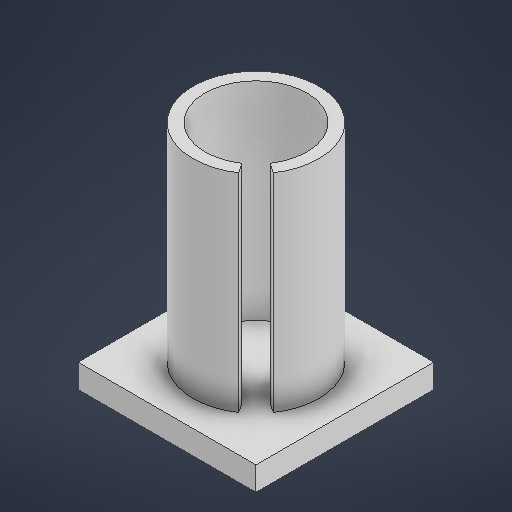
# Autodesk Inventor part: Część1
Saved by Autodesk Inventor 2026 (Build 300175050, 175E)
## iProperties
Created: 2026-01-10
Part Number: Część1
Material: Ogólny
Document SubType Name: Modeling
Designer: DeathLock
Density: 1 g/cm^3
Appearance: Domyślna
Author: DeathLock
Autodesk Inventor part; units mm, degrees
ref_plane "YZ Plane" through (0, 0, 0) normal (1, 0, 0) x (0, 1, 0)
ref_plane "XZ Plane" through (0, 0, 0) normal (0, 1, 0) x (-1, 0, 0)
ref_plane "XY Plane" through (0, 0, 0) normal (0, 0, 1) x (1, 0, 0)
sketch "Szkic1" plane through (0, 0, 0) normal (0, 1, 0) x (-1, 0, 0)
  line L0 (1.4259, 1.5074) -> (-13.5741, 1.5074)
  line L1 (-13.5741, 1.5074) -> (-13.5741, -13.4926)
  line L2 (-13.5741, -13.4926) -> (1.4259, -13.4926)
  line L3 (1.4259, -13.4926) -> (1.4259, 1.5074)
  point P0 (0, 0)
  dimension "d0" = 15
  dimension "d1" = 15
  constraints: 8 end point, 2 parallel, 1 horizontal, 1 perpendicular
  measures "d0" distance of L2.end L1.end
  measures "d1" distance of L1.end L0.end
extrude "Wyciągnięcie proste1" add sketch "Szkic1" along normal blind 2
sketch "Szkic2" plane through (0, 2, 0) normal (0, 1, 0) x (1, 0, 0)
  line L0 (-1.4259, 13.4926) -> (-1.4259, -1.5074) projected
  line L1 (-1.4259, 5.9926) -> (13.5741, 5.9926)
  line L2 (13.5741, -1.5074) -> (13.5741, 13.4926) projected
  line L3 (-1.4259, -1.5074) -> (13.5741, -1.5074) projected
  line L4 (6.0741, -1.5074) -> (6.0741, 5.9926)
  circle A0 centre (6.0741, 5.9926) radius 4.3
  circle A1 centre (6.0741, 5.9926) radius 5.3
  line L5 (6.0741, 5.9926) -> (9.1146, 2.952)
  line L6 (6.0741, 5.9926) -> (10.3741, 5.9926) construction
  line L7 (6.0741, 5.9926) -> (7.7196, 2.0199)
  line L8 (6.0741, 5.9926) -> (10.3741, 5.9926) construction
  line L9 (6.0741, 5.9926) -> (10.0468, 4.347)
  line L10 (6.0741, 5.9926) -> (10.3741, 5.9926) construction
  line L11 (10.0468, 4.347) -> (10.9706, 3.9644)
  line L12 (7.7196, 2.0199) -> (8.1023, 1.096)
  line L13 (6.0741, 5.9926) -> (8.463, 2.4173)
  line L14 (6.0741, 5.9926) -> (10.3741, 5.9926) construction
  line L15 (8.463, 2.4173) -> (9.0186, 1.5858)
  line L16 (6.0741, 5.9926) -> (9.6494, 3.6036)
  line L17 (6.0741, 5.9926) -> (10.3741, 5.9926) construction
  line L18 (9.6494, 3.6036) -> (10.4809, 3.0481)
  point P0 (0, 0)
  dimension "d4" = 8.6
  dimension "d5" = 10.6
  dimension "d6" = 45
  dimension "d7" = 67.5
  dimension "d8" = 22.5
  dimension "d14" = 56.25
  dimension "d15" = 4.3
  dimension "d16" = 33.75
  constraints: 32 end point, 8 point on circle, 5 equal length, 5 horizontal, 4 midpoint, 2 centre point, 2 coincident, 2 point on line
  measures "d4" diameter of A0
  measures "d5" diameter of A1
  measures "d6" angle of L5 L6
  measures "d7" angle of L7 L8
  measures "d8" angle of L9 L10
  measures "d14" angle of L13 L14
  measures "d15" distance of L5.start L16.end
  measures "d16" angle of L16 L17
extrude "Wyciągnięcie proste2" add sketch "Szkic2" along normal blind 17.5 contours A1 L1 A0 | L1 A0 L4 A1 | A1 L11 A0 L1 | L4 A0 L12 A1 | A1 L18 A0 L11 | L12 A0 L15 A1
